side_short_v19 (Autodesk Fusion 360 design; units mm, degrees)
Autodesk Fusion 360 part; units mm, degrees
sketch "Sketch1" plane through (0, 0, 0) normal (1, 0, 0) x (0, 0, -1)
  line L0 (0, 0) -> (226.726, 0)
  line L1 (226.726, 0) -> (226.726, 70.4)
  line L2 (226.726, 70.4) -> (0, 70.4)
  line L3 (0, 70.4) -> (0, 0)
  line L4 (5.4, 0) -> (25.3, 0)
  line L5 (25.3, 0) -> (25.3, 32.4)
  line L6 (25.3, 32.4) -> (5.4, 32.4)
  line L7 (5.4, 32.4) -> (5.4, 0)
  line L8 (103.413, 0) -> (123.313, 0)
  line L9 (123.313, 0) -> (123.313, 32.4)
  line L10 (123.313, 32.4) -> (103.413, 32.4)
  line L11 (103.413, 32.4) -> (103.413, 0)
  line L12 (221.326, 0) -> (201.426, 0)
  line L13 (201.426, 0) -> (201.426, 32.4)
  line L14 (201.426, 32.4) -> (221.326, 32.4)
  line L15 (221.326, 32.4) -> (221.326, 0)
  dimension "d1" = 226.726
  dimension "d2" = 70.4
  dimension "d3" = 19.9
  dimension "d4" = 19.9
  dimension "d5" = 19.9
  dimension "d6" = 5.4
  dimension "d7" = 5.4
  dimension "d8" = 32.4
  dimension "d9" = 32.4
  dimension "d10" = 32.4
  dimension "d11" = 103.413
  constraint horizontal L0
  constraint vertical L1
  constraint horizontal L2
  constraint vertical L3
  constraint coincident L0.start L3.end
  constraint horizontal L4
  constraint vertical L5
  constraint horizontal L6
  constraint vertical L7
  constraint coincident L0 L4.start
  constraint horizontal L8
  constraint vertical L9
  constraint horizontal L10
  constraint vertical L11
  constraint coincident L0 L8.start
  constraint horizontal L12
  constraint vertical L13
  constraint horizontal L14
  constraint vertical L15
  constraint coincident L0 L12.start
  measures "d1" distance of L0.start L0.end
  measures "d2" distance of L0.start L2.end
  measures "d3" distance of L5.end L6.end
  measures "d4" distance of L9.end L10.end
  measures "d5" distance of L13.end L14.end
  measures "d6" distance of L3 L7
  measures "d7" distance of L1 L15
  measures "d8" distance of L4.start L6.end
  measures "d9" distance of L8.start L10.end
  measures "d10" distance of L12.end L13.end
  measures "d11" distance of L1 L9
extrude "Extrude1" add sketch "Sketch1" along normal blind 5.4 contours L0 L1 L2 L3 L5 L6 L7 L9 L10 L11 L13 L14 L15
sketch "Sketch2" plane through (5.4, 0, 0) normal (1, 0, 0) x (0, 0, -1)
  line L0 (123.313, 0) -> (201.426, 0)
  line L1 (201.426, 0) -> (201.426, 32.4)
  line L2 (201.426, 32.4) -> (221.326, 32.4)
  line L3 (221.326, 32.4) -> (221.326, 0)
  line L4 (221.326, 0) -> (226.726, 0)
  line L5 (226.726, 0) -> (226.726, 70.4)
  line L6 (226.726, 70.4) -> (0, 70.4)
  line L7 (0, 70.4) -> (0, 0)
  line L8 (0, 0) -> (5.4, 0)
  line L9 (5.4, 0) -> (5.4, 32.4)
  line L10 (5.4, 32.4) -> (25.3, 32.4)
  line L11 (25.3, 32.4) -> (25.3, 0)
  line L12 (25.3, 0) -> (103.413, 0)
  line L13 (103.413, 0) -> (103.413, 32.4)
  line L14 (103.413, 32.4) -> (123.313, 32.4)
  line L15 (123.313, 32.4) -> (123.313, 0)
  line L16 (153.363, 32.4) -> (73.363, 32.4)
  arc A0 (73.363, 32.4) -> (73.363, 22.4) centre (73.363, 27.4) ccw
  line L17 (73.363, 22.4) -> (153.363, 22.4)
  arc A1 (153.363, 22.4) -> (153.363, 32.4) centre (153.363, 27.4) ccw
  line L18 (153.363, 27.4) -> (73.363, 27.4) construction
  point P0 (113.363, 27.4)
  dimension "d14" = 5
  dimension "d15" = 80
  dimension "d16" = 226.726
  dimension "d17" = 113.363
  constraint tangent L16 A0
  constraint tangent A0 L17
  constraint parallel L16 L17
  constraint tangent L17 A1
  constraint tangent L16 A1
  constraint perpendicular L13 L18
  constraint midpoint L18 P0
  constraint collinear L14 L16
  measures "d14" radius of A0
  measures "d15" distance of A1.centre A0.centre
  measures "d16" distance of L5.end L6.end
  measures "d17" distance of L7 P0
extrude "Extrude2" cut sketch "Sketch2" against normal blind 10 contours L15 L16 L17 A1 | L13 L16 A0 L17
sketch "export" plane through (5.4, 0, 0) normal (1, 0, 0) x (0, 0, -1)
  line L0 (103.413, 22.4) -> (73.363, 22.4)
  arc A0 (73.363, 32.4) -> (73.363, 22.4) centre (73.363, 27.4) ccw
  line L1 (73.363, 32.4) -> (153.363, 32.4)
  arc A1 (153.363, 22.4) -> (153.363, 32.4) centre (153.363, 27.4) ccw
  line L2 (153.363, 22.4) -> (123.313, 22.4)
  line L3 (123.313, 22.4) -> (123.313, 0)
  line L4 (123.313, 0) -> (201.426, 0)
  line L5 (201.426, 0) -> (201.426, 32.4)
  line L6 (201.426, 32.4) -> (221.326, 32.4)
  line L7 (221.326, 32.4) -> (221.326, 0)
  line L8 (221.326, 0) -> (226.726, 0)
  line L9 (226.726, 0) -> (226.726, 70.4)
  line L10 (226.726, 70.4) -> (0, 70.4)
  line L11 (0, 70.4) -> (0, 0)
  line L12 (0, 0) -> (5.4, 0)
  line L13 (5.4, 0) -> (5.4, 32.4)
  line L14 (5.4, 32.4) -> (25.3, 32.4)
  line L15 (25.3, 32.4) -> (25.3, 0)
  line L16 (25.3, 0) -> (103.413, 0)
  line L17 (103.413, 0) -> (103.413, 22.4)
equation "d2 = d8 + 38 mm"
equation "d4 = d3"
equation "d5 = d4"
equation "d7 = d6"
equation "d8 = 6 * 5.4 mm"
equation "d9 = d8"
equation "d10 = d9"
equation "d11 = ( d1 - d4 ) / 2"
equation "d17 = d16 / 2"
